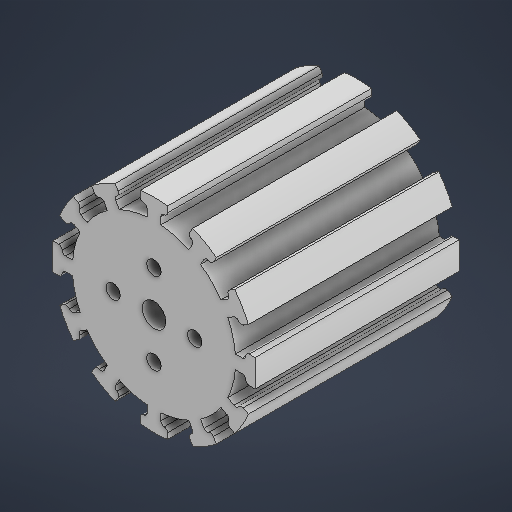
# Autodesk Inventor part: внутр сиськи
Saved by Autodesk Inventor 2025 (Build 290162000, 162)
## iProperties
Created: 2025-11-06
Part Number: внутр сиськи
Material: Типовые
Document SubType Name: Modeling
Designer: Phantom
Density: 1 g/cm^3
Appearance: По умолчанию
Author: Phantom
Autodesk Inventor part; units mm, degrees
ref_plane "YZ Plane" through (0, 0, 0) normal (1, 0, 0) x (0, 1, 0)
ref_plane "XZ Plane" through (0, 0, 0) normal (0, 1, 0) x (-1, 0, 0)
ref_plane "XY Plane" through (0, 0, 0) normal (0, 0, 1) x (1, 0, 0)
sketch "Эскиз1" plane through (0, 0, 0) normal (0, 0, 1) x (1, 0, 0)
  arc A0 (25.6449, 2.3551) -> (26.6449, 3.3551) centre (25.6449, 3.3551) ccw
  arc A1 (27.6449, 4.3551) -> (26.6449, 3.3551) centre (27.6449, 3.3551) ccw
  line L0 (27.6449, 4.3551) -> (29.3771, 4.3551)
  arc A2 (29.3771, -3.6449) -> (29.3771, 4.3551) centre (-0.3551, 0.3551) ccw
  line L1 (29.3771, -3.6449) -> (27.6449, -3.6449)
  arc A3 (26.6449, -2.6449) -> (27.6449, -3.6449) centre (27.6449, -2.6449) ccw
  arc A4 (26.6449, -2.6449) -> (25.6449, -1.6449) centre (25.6449, -2.6449) ccw
  line L2 (25.6449, -1.6449) -> (23.5615, -1.6449)
  arc A5 (21.3572, -9.8711) -> (23.5615, -1.6449) centre (-0.3551, 0.3551) ccw
  line L3 (21.3572, -9.8711) -> (23.1616, -10.9129)
  arc A6 (23.1616, -10.9129) -> (24.5276, -10.5469) centre (23.6616, -10.0469) ccw
  arc A7 (25.8936, -10.1808) -> (24.5276, -10.5469) centre (25.3936, -11.0469) ccw
  line L4 (25.8936, -10.1808) -> (27.3937, -11.0469)
  arc A8 (23.3937, -17.9751) -> (27.3937, -11.0469) centre (-0.3551, 0.3551) ccw
  line L5 (23.3937, -17.9751) -> (21.8936, -17.109)
  arc A9 (21.5276, -15.743) -> (21.8936, -17.109) centre (22.3936, -16.243) ccw
  arc A10 (21.5276, -15.743) -> (21.1616, -14.377) centre (20.6616, -15.243) ccw
  line L6 (21.1616, -14.377) -> (19.3572, -13.3352)
  arc A11 (13.3352, -19.3572) -> (19.3572, -13.3352) centre (-0.3551, 0.3551) ccw
  line L7 (13.3352, -19.3572) -> (14.377, -21.1616)
  arc A12 (14.377, -21.1616) -> (15.743, -21.5276) centre (15.243, -20.6616) ccw
  arc A13 (17.109, -21.8936) -> (15.743, -21.5276) centre (16.243, -22.3936) ccw
  line L8 (17.109, -21.8936) -> (17.9751, -23.3937)
  arc A14 (11.0469, -27.3937) -> (17.9751, -23.3937) centre (-0.3551, 0.3551) ccw
  line L9 (11.0469, -27.3937) -> (10.1808, -25.8936)
  arc A15 (10.5469, -24.5276) -> (10.1808, -25.8936) centre (11.0469, -25.3936) ccw
  arc A16 (10.5469, -24.5276) -> (10.9129, -23.1616) centre (10.0469, -23.6616) ccw
  line L10 (10.9129, -23.1616) -> (9.8711, -21.3572)
  arc A17 (1.6449, -23.5615) -> (9.8711, -21.3572) centre (-0.3551, 0.3551) ccw
  line L11 (1.6449, -23.5615) -> (1.6449, -25.6449)
  arc A18 (1.6449, -25.6449) -> (2.6449, -26.6449) centre (2.6449, -25.6449) ccw
  arc A19 (3.6449, -27.6449) -> (2.6449, -26.6449) centre (2.6449, -27.6449) ccw
  line L12 (3.6449, -27.6449) -> (3.6449, -29.3771)
  arc A20 (-4.3551, -29.3771) -> (3.6449, -29.3771) centre (-0.3551, 0.3551) ccw
  line L13 (-4.3551, -29.3771) -> (-4.3551, -27.6449)
  arc A21 (-3.3551, -26.6449) -> (-4.3551, -27.6449) centre (-3.3551, -27.6449) ccw
  arc A22 (-3.3551, -26.6449) -> (-2.3551, -25.6449) centre (-3.3551, -25.6449) ccw
  line L14 (-2.3551, -25.6449) -> (-2.3551, -23.5615)
  arc A23 (-10.5813, -21.3572) -> (-2.3551, -23.5615) centre (-0.3551, 0.3551) ccw
  line L15 (-10.5813, -21.3572) -> (-11.623, -23.1616)
  arc A24 (-11.623, -23.1616) -> (-11.257, -24.5276) centre (-10.757, -23.6616) ccw
  arc A25 (-10.891, -25.8936) -> (-11.257, -24.5276) centre (-11.757, -25.3936) ccw
  line L16 (-10.891, -25.8936) -> (-11.757, -27.3937)
  arc A26 (-18.6852, -23.3937) -> (-11.757, -27.3937) centre (-0.3551, 0.3551) ccw
  line L17 (-18.6852, -23.3937) -> (-17.8192, -21.8936)
  arc A27 (-16.4531, -21.5276) -> (-17.8192, -21.8936) centre (-16.9531, -22.3936) ccw
  arc A28 (-16.4531, -21.5276) -> (-15.0871, -21.1616) centre (-15.9531, -20.6616) ccw
  line L18 (-15.0871, -21.1616) -> (-14.0454, -19.3572)
  arc A29 (-20.0674, -13.3352) -> (-14.0454, -19.3572) centre (-0.3551, 0.3551) ccw
  line L19 (-20.0674, -13.3352) -> (-21.8717, -14.377)
  arc A30 (-21.8717, -14.377) -> (-22.2378, -15.743) centre (-21.3717, -15.243) ccw
  arc A31 (-22.6038, -17.109) -> (-22.2378, -15.743) centre (-23.1038, -16.243) ccw
  line L20 (-22.6038, -17.109) -> (-24.1039, -17.9751)
  arc A32 (-28.1039, -11.0469) -> (-24.1039, -17.9751) centre (-0.3551, 0.3551) ccw
  line L21 (-28.1039, -11.0469) -> (-26.6038, -10.1808)
  arc A33 (-25.2378, -10.5469) -> (-26.6038, -10.1808) centre (-26.1038, -11.0469) ccw
  arc A34 (-25.2378, -10.5469) -> (-23.8717, -10.9129) centre (-24.3717, -10.0469) ccw
  line L22 (-23.8717, -10.9129) -> (-22.0674, -9.8711)
  arc A35 (-24.2716, -1.6449) -> (-22.0674, -9.8711) centre (-0.3551, 0.3551) ccw
  line L23 (-24.2716, -1.6449) -> (-26.3551, -1.6449)
  arc A36 (-26.3551, -1.6449) -> (-27.3551, -2.6449) centre (-26.3551, -2.6449) ccw
  arc A37 (-28.3551, -3.6449) -> (-27.3551, -2.6449) centre (-28.3551, -2.6449) ccw
  line L24 (-28.3551, -3.6449) -> (-30.0872, -3.6449)
  arc A38 (-30.0872, 4.3551) -> (-30.0872, -3.6449) centre (-0.3551, 0.3551) ccw
  line L25 (-30.0872, 4.3551) -> (-28.3551, 4.3551)
  arc A39 (-27.3551, 3.3551) -> (-28.3551, 4.3551) centre (-28.3551, 3.3551) ccw
  arc A40 (-27.3551, 3.3551) -> (-26.3551, 2.3551) centre (-26.3551, 3.3551) ccw
  line L26 (-26.3551, 2.3551) -> (-24.2716, 2.3551)
  arc A41 (-22.0674, 10.5813) -> (-24.2716, 2.3551) centre (-0.3551, 0.3551) ccw
  line L27 (-22.0674, 10.5813) -> (-23.8717, 11.623)
  arc A42 (-23.8717, 11.623) -> (-25.2378, 11.257) centre (-24.3717, 10.757) ccw
  arc A43 (-26.6038, 10.891) -> (-25.2378, 11.257) centre (-26.1038, 11.757) ccw
  line L28 (-26.6038, 10.891) -> (-28.1039, 11.757)
  arc A44 (-24.1039, 18.6852) -> (-28.1039, 11.757) centre (-0.3551, 0.3551) ccw
  line L29 (-24.1039, 18.6852) -> (-22.6038, 17.8192)
  arc A45 (-22.2378, 16.4531) -> (-22.6038, 17.8192) centre (-23.1038, 16.9531) ccw
  arc A46 (-22.2378, 16.4531) -> (-21.8717, 15.0871) centre (-21.3717, 15.9531) ccw
  line L30 (-21.8717, 15.0871) -> (-20.0674, 14.0454)
  arc A47 (-14.0454, 20.0674) -> (-20.0674, 14.0454) centre (-0.3551, 0.3551) ccw
  line L31 (-14.0454, 20.0674) -> (-15.0871, 21.8717)
  arc A48 (-15.0871, 21.8717) -> (-16.4531, 22.2378) centre (-15.9531, 21.3717) ccw
  arc A49 (-17.8192, 22.6038) -> (-16.4531, 22.2378) centre (-16.9531, 23.1038) ccw
  line L32 (-17.8192, 22.6038) -> (-18.6852, 24.1039)
  arc A50 (-11.757, 28.1039) -> (-18.6852, 24.1039) centre (-0.3551, 0.3551) ccw
  line L33 (-11.757, 28.1039) -> (-10.891, 26.6038)
  arc A51 (-11.257, 25.2378) -> (-10.891, 26.6038) centre (-11.757, 26.1038) ccw
  arc A52 (-11.257, 25.2378) -> (-11.623, 23.8717) centre (-10.757, 24.3717) ccw
  line L34 (-11.623, 23.8717) -> (-10.5813, 22.0674)
  arc A53 (-2.3551, 24.2716) -> (-10.5813, 22.0674) centre (-0.3551, 0.3551) ccw
  line L35 (-2.3551, 24.2716) -> (-2.3551, 26.3551)
  arc A54 (-2.3551, 26.3551) -> (-3.3551, 27.3551) centre (-3.3551, 26.3551) ccw
  arc A55 (-4.3551, 28.3551) -> (-3.3551, 27.3551) centre (-3.3551, 28.3551) ccw
  line L36 (-4.3551, 28.3551) -> (-4.3551, 30.0872)
  arc A56 (3.6449, 30.0872) -> (-4.3551, 30.0872) centre (-0.3551, 0.3551) ccw
  line L37 (3.6449, 30.0872) -> (3.6449, 28.3551)
  arc A57 (2.6449, 27.3551) -> (3.6449, 28.3551) centre (2.6449, 28.3551) ccw
  arc A58 (2.6449, 27.3551) -> (1.6449, 26.3551) centre (2.6449, 26.3551) ccw
  line L38 (1.6449, 26.3551) -> (1.6449, 24.2716)
  arc A59 (9.8711, 22.0674) -> (1.6449, 24.2716) centre (-0.3551, 0.3551) ccw
  line L39 (9.8711, 22.0674) -> (10.9129, 23.8717)
  arc A60 (10.9129, 23.8717) -> (10.5469, 25.2378) centre (10.0469, 24.3717) ccw
  arc A61 (10.1808, 26.6038) -> (10.5469, 25.2378) centre (11.0469, 26.1038) ccw
  line L40 (10.1808, 26.6038) -> (11.0469, 28.1039)
  arc A62 (17.9751, 24.1039) -> (11.0469, 28.1039) centre (-0.3551, 0.3551) ccw
  line L41 (17.9751, 24.1039) -> (17.109, 22.6038)
  arc A63 (15.743, 22.2378) -> (17.109, 22.6038) centre (16.243, 23.1038) ccw
  arc A64 (15.743, 22.2378) -> (14.377, 21.8717) centre (15.243, 21.3717) ccw
  line L42 (14.377, 21.8717) -> (13.3352, 20.0674)
  arc A65 (19.3572, 14.0454) -> (13.3352, 20.0674) centre (-0.3551, 0.3551) ccw
  line L43 (19.3572, 14.0454) -> (21.1616, 15.0871)
  arc A66 (21.1616, 15.0871) -> (21.5276, 16.4531) centre (20.6616, 15.9531) ccw
  arc A67 (21.8936, 17.8192) -> (21.5276, 16.4531) centre (22.3936, 16.9531) ccw
  line L44 (21.8936, 17.8192) -> (23.3937, 18.6852)
  arc A68 (27.3937, 11.757) -> (23.3937, 18.6852) centre (-0.3551, 0.3551) ccw
  line L45 (27.3937, 11.757) -> (25.8936, 10.891)
  arc A69 (24.5276, 11.257) -> (25.8936, 10.891) centre (25.3936, 11.757) ccw
  arc A70 (24.5276, 11.257) -> (23.1616, 11.623) centre (23.6616, 10.757) ccw
  line L46 (23.1616, 11.623) -> (21.3572, 10.5813)
  arc A71 (23.5615, 2.3551) -> (21.3572, 10.5813) centre (-0.3551, 0.3551) ccw
  line L47 (23.5615, 2.3551) -> (25.6449, 2.3551)
  circle A72 centre (-0.3551, 0.3551) radius 3.5
  circle A73 centre (-0.3551, 0.3551) radius 12
  circle A74 centre (-0.3551, 12.3551) radius 4.5
  circle A75 centre (-12.3551, 0.3551) radius 4.5
  circle A76 centre (-0.3551, -11.6449) radius 4.5
  circle A77 centre (11.6449, 0.3551) radius 4.5
  point P0 (0, 0)
  point P1 (-0.3619, 0.2649)
  point P2 (0, 0.7101)
  point P3 (-0.7101, 0.7101)
  point P4 (-0.7101, 0)
  dimension "d1" = 24
  dimension "d0" = 7
  dimension "d2" = 9
  dimension "d5" = 360
  constraints: 144 point on circle, 96 end point, 77 centre point, 2 coincident, 1 vertical alignment, 15 other
  measures "d0" diameter of A72
  measures "d2" diameter of A74
extrude "Выдавливание1" add sketch "Эскиз1" along normal blind 60 contours A0 A1 L0 A2 L1 A3 A4 L2 A5 L3 A6 A7 L4 A8 L5 A9 A10 L6 A11 L7 A12 A13 L8 A14 L9 A15 A16 L10 A17 L11 A18 A19 L12 A20 L13 A21 A22 L14 A23 L15 A24 A25 L16 A26 L17 A27 A28 L18 A29 L19 A30 A31 L20 A32 L21 A33 A34 L22 A35 L23 A36 A37 L24 A38 L25 A39 A40 L26 A41 L27 A42 A43 L28 A44 L29 A45 A46 L30 A47 L31 A48 A49 L32 A50 L33 A51 A52 L34 A53 L35 A54 A55 L36 A56 L37 A57 A58 L38 A59 L39 A60 A61 L40 A62 L41 A63 A64 L42 A65 L43 A66 A67 L44 A68 L45 A69 A70 L46 A71 L47 | A77 A73 A76 A75 A74
sketch "Эскиз2" plane through (0, 0, 60) normal (0, 0, 1) x (1, 0, 0)
  line L0 (-4.3551, -27.6449) -> (-4.3551, -29.3771) projected
  arc A0 (-4.3551, -29.3771) -> (3.6449, -29.3771) centre (-0.3551, 0.3551) ccw projected
  line L1 (3.6449, -29.3771) -> (3.6449, -27.6449) projected
  arc A1 (3.6449, -27.6449) -> (2.6449, -26.6449) centre (2.6449, -27.6449) ccw projected
  arc A2 (1.6449, -25.6449) -> (2.6449, -26.6449) centre (2.6449, -25.6449) ccw projected
  line L2 (1.6449, -25.6449) -> (1.6449, -23.5615) projected
  arc A3 (1.6449, -23.5615) -> (9.8711, -21.3572) centre (-0.3551, 0.3551) ccw projected
  line L3 (9.8711, -21.3572) -> (10.9129, -23.1616) projected
  arc A4 (10.5469, -24.5276) -> (10.9129, -23.1616) centre (10.0469, -23.6616) ccw projected
  arc A5 (10.5469, -24.5276) -> (10.1808, -25.8936) centre (11.0469, -25.3936) ccw projected
  line L4 (10.1808, -25.8936) -> (11.0469, -27.3937) projected
  arc A6 (11.0469, -27.3937) -> (17.9751, -23.3937) centre (-0.3551, 0.3551) ccw projected
  line L5 (17.9751, -23.3937) -> (17.109, -21.8936) projected
  arc A7 (17.109, -21.8936) -> (15.743, -21.5276) centre (16.243, -22.3936) ccw projected
  arc A8 (14.377, -21.1616) -> (15.743, -21.5276) centre (15.243, -20.6616) ccw projected
  line L6 (14.377, -21.1616) -> (13.3352, -19.3572) projected
  arc A9 (13.3352, -19.3572) -> (19.3572, -13.3352) centre (-0.3551, 0.3551) ccw projected
  line L7 (19.3572, -13.3352) -> (21.1616, -14.377) projected
  arc A10 (21.5276, -15.743) -> (21.1616, -14.377) centre (20.6616, -15.243) ccw projected
  arc A11 (21.5276, -15.743) -> (21.8936, -17.109) centre (22.3936, -16.243) ccw projected
  line L8 (21.8936, -17.109) -> (23.3937, -17.9751) projected
  arc A12 (23.3937, -17.9751) -> (27.3937, -11.0469) centre (-0.3551, 0.3551) ccw projected
  line L9 (27.3937, -11.0469) -> (25.8936, -10.1808) projected
  arc A13 (25.8936, -10.1808) -> (24.5276, -10.5469) centre (25.3936, -11.0469) ccw projected
  arc A14 (23.1616, -10.9129) -> (24.5276, -10.5469) centre (23.6616, -10.0469) ccw projected
  line L10 (23.1616, -10.9129) -> (21.3572, -9.8711) projected
  arc A15 (21.3572, -9.8711) -> (23.5615, -1.6449) centre (-0.3551, 0.3551) ccw projected
  line L11 (23.5615, -1.6449) -> (25.6449, -1.6449) projected
  arc A16 (26.6449, -2.6449) -> (25.6449, -1.6449) centre (25.6449, -2.6449) ccw projected
  arc A17 (26.6449, -2.6449) -> (27.6449, -3.6449) centre (27.6449, -2.6449) ccw projected
  line L12 (27.6449, -3.6449) -> (29.3771, -3.6449) projected
  arc A18 (29.3771, -3.6449) -> (29.3771, 4.3551) centre (-0.3551, 0.3551) ccw projected
  line L13 (29.3771, 4.3551) -> (27.6449, 4.3551) projected
  arc A19 (27.6449, 4.3551) -> (26.6449, 3.3551) centre (27.6449, 3.3551) ccw projected
  arc A20 (25.6449, 2.3551) -> (26.6449, 3.3551) centre (25.6449, 3.3551) ccw projected
  line L14 (25.6449, 2.3551) -> (23.5615, 2.3551) projected
  arc A21 (23.5615, 2.3551) -> (21.3572, 10.5813) centre (-0.3551, 0.3551) ccw projected
  line L15 (21.3572, 10.5813) -> (23.1616, 11.623) projected
  arc A22 (24.5276, 11.257) -> (23.1616, 11.623) centre (23.6616, 10.757) ccw projected
  arc A23 (24.5276, 11.257) -> (25.8936, 10.891) centre (25.3936, 11.757) ccw projected
  line L16 (25.8936, 10.891) -> (27.3937, 11.757) projected
  arc A24 (27.3937, 11.757) -> (23.3937, 18.6852) centre (-0.3551, 0.3551) ccw projected
  line L17 (23.3937, 18.6852) -> (21.8936, 17.8192) projected
  arc A25 (21.8936, 17.8192) -> (21.5276, 16.4531) centre (22.3936, 16.9531) ccw projected
  arc A26 (21.1616, 15.0871) -> (21.5276, 16.4531) centre (20.6616, 15.9531) ccw projected
  line L18 (21.1616, 15.0871) -> (19.3572, 14.0454) projected
  arc A27 (19.3572, 14.0454) -> (13.3352, 20.0674) centre (-0.3551, 0.3551) ccw projected
  line L19 (13.3352, 20.0674) -> (14.377, 21.8717) projected
  arc A28 (15.743, 22.2378) -> (14.377, 21.8717) centre (15.243, 21.3717) ccw projected
  arc A29 (15.743, 22.2378) -> (17.109, 22.6038) centre (16.243, 23.1038) ccw projected
  line L20 (17.109, 22.6038) -> (17.9751, 24.1039) projected
  arc A30 (17.9751, 24.1039) -> (11.0469, 28.1039) centre (-0.3551, 0.3551) ccw projected
  line L21 (11.0469, 28.1039) -> (10.1808, 26.6038) projected
  arc A31 (10.1808, 26.6038) -> (10.5469, 25.2378) centre (11.0469, 26.1038) ccw projected
  arc A32 (10.9129, 23.8717) -> (10.5469, 25.2378) centre (10.0469, 24.3717) ccw projected
  line L22 (10.9129, 23.8717) -> (9.8711, 22.0674) projected
  arc A33 (9.8711, 22.0674) -> (1.6449, 24.2716) centre (-0.3551, 0.3551) ccw projected
  line L23 (1.6449, 24.2716) -> (1.6449, 26.3551) projected
  arc A34 (2.6449, 27.3551) -> (1.6449, 26.3551) centre (2.6449, 26.3551) ccw projected
  arc A35 (2.6449, 27.3551) -> (3.6449, 28.3551) centre (2.6449, 28.3551) ccw projected
  line L24 (3.6449, 28.3551) -> (3.6449, 30.0872) projected
  arc A36 (3.6449, 30.0872) -> (-4.3551, 30.0872) centre (-0.3551, 0.3551) ccw projected
  line L25 (-4.3551, 30.0872) -> (-4.3551, 28.3551) projected
  arc A37 (-4.3551, 28.3551) -> (-3.3551, 27.3551) centre (-3.3551, 28.3551) ccw projected
  arc A38 (-2.3551, 26.3551) -> (-3.3551, 27.3551) centre (-3.3551, 26.3551) ccw projected
  line L26 (-2.3551, 26.3551) -> (-2.3551, 24.2716) projected
  arc A39 (-2.3551, 24.2716) -> (-10.5813, 22.0674) centre (-0.3551, 0.3551) ccw projected
  line L27 (-10.5813, 22.0674) -> (-11.623, 23.8717) projected
  arc A40 (-11.257, 25.2378) -> (-11.623, 23.8717) centre (-10.757, 24.3717) ccw projected
  arc A41 (-11.257, 25.2378) -> (-10.891, 26.6038) centre (-11.757, 26.1038) ccw projected
  line L28 (-10.891, 26.6038) -> (-11.757, 28.1039) projected
  arc A42 (-11.757, 28.1039) -> (-18.6852, 24.1039) centre (-0.3551, 0.3551) ccw projected
  line L29 (-18.6852, 24.1039) -> (-17.8192, 22.6038) projected
  arc A43 (-17.8192, 22.6038) -> (-16.4531, 22.2378) centre (-16.9531, 23.1038) ccw projected
  arc A44 (-15.0871, 21.8717) -> (-16.4531, 22.2378) centre (-15.9531, 21.3717) ccw projected
  line L30 (-15.0871, 21.8717) -> (-14.0454, 20.0674) projected
  arc A45 (-14.0454, 20.0674) -> (-20.0674, 14.0454) centre (-0.3551, 0.3551) ccw projected
  line L31 (-20.0674, 14.0454) -> (-21.8717, 15.0871) projected
  arc A46 (-22.2378, 16.4531) -> (-21.8717, 15.0871) centre (-21.3717, 15.9531) ccw projected
  arc A47 (-22.2378, 16.4531) -> (-22.6038, 17.8192) centre (-23.1038, 16.9531) ccw projected
  line L32 (-22.6038, 17.8192) -> (-24.1039, 18.6852) projected
  arc A48 (-24.1039, 18.6852) -> (-28.1039, 11.757) centre (-0.3551, 0.3551) ccw projected
  line L33 (-28.1039, 11.757) -> (-26.6038, 10.891) projected
  arc A49 (-26.6038, 10.891) -> (-25.2378, 11.257) centre (-26.1038, 11.757) ccw projected
  arc A50 (-23.8717, 11.623) -> (-25.2378, 11.257) centre (-24.3717, 10.757) ccw projected
  line L34 (-23.8717, 11.623) -> (-22.0674, 10.5813) projected
  arc A51 (-22.0674, 10.5813) -> (-24.2716, 2.3551) centre (-0.3551, 0.3551) ccw projected
  line L35 (-24.2716, 2.3551) -> (-26.3551, 2.3551) projected
  arc A52 (-27.3551, 3.3551) -> (-26.3551, 2.3551) centre (-26.3551, 3.3551) ccw projected
  arc A53 (-27.3551, 3.3551) -> (-28.3551, 4.3551) centre (-28.3551, 3.3551) ccw projected
  line L36 (-28.3551, 4.3551) -> (-30.0872, 4.3551) projected
  arc A54 (-30.0872, 4.3551) -> (-30.0872, -3.6449) centre (-0.3551, 0.3551) ccw projected
  line L37 (-30.0872, -3.6449) -> (-28.3551, -3.6449) projected
  arc A55 (-28.3551, -3.6449) -> (-27.3551, -2.6449) centre (-28.3551, -2.6449) ccw projected
  arc A56 (-26.3551, -1.6449) -> (-27.3551, -2.6449) centre (-26.3551, -2.6449) ccw projected
  line L38 (-26.3551, -1.6449) -> (-24.2716, -1.6449) projected
  arc A57 (-24.2716, -1.6449) -> (-22.0674, -9.8711) centre (-0.3551, 0.3551) ccw projected
  line L39 (-22.0674, -9.8711) -> (-23.8717, -10.9129) projected
  arc A58 (-25.2378, -10.5469) -> (-23.8717, -10.9129) centre (-24.3717, -10.0469) ccw projected
  arc A59 (-25.2378, -10.5469) -> (-26.6038, -10.1808) centre (-26.1038, -11.0469) ccw projected
  line L40 (-26.6038, -10.1808) -> (-28.1039, -11.0469) projected
  arc A60 (-28.1039, -11.0469) -> (-24.1039, -17.9751) centre (-0.3551, 0.3551) ccw projected
  line L41 (-24.1039, -17.9751) -> (-22.6038, -17.109) projected
  arc A61 (-22.6038, -17.109) -> (-22.2378, -15.743) centre (-23.1038, -16.243) ccw projected
  arc A62 (-21.8717, -14.377) -> (-22.2378, -15.743) centre (-21.3717, -15.243) ccw projected
  line L42 (-21.8717, -14.377) -> (-20.0674, -13.3352) projected
  arc A63 (-20.0674, -13.3352) -> (-14.0454, -19.3572) centre (-0.3551, 0.3551) ccw projected
  line L43 (-14.0454, -19.3572) -> (-15.0871, -21.1616) projected
  arc A64 (-16.4531, -21.5276) -> (-15.0871, -21.1616) centre (-15.9531, -20.6616) ccw projected
  arc A65 (-16.4531, -21.5276) -> (-17.8192, -21.8936) centre (-16.9531, -22.3936) ccw projected
  line L44 (-17.8192, -21.8936) -> (-18.6852, -23.3937) projected
  arc A66 (-18.6852, -23.3937) -> (-11.757, -27.3937) centre (-0.3551, 0.3551) ccw projected
  line L45 (-11.757, -27.3937) -> (-10.891, -25.8936) projected
  arc A67 (-10.891, -25.8936) -> (-11.257, -24.5276) centre (-11.757, -25.3936) ccw projected
  arc A68 (-11.623, -23.1616) -> (-11.257, -24.5276) centre (-10.757, -23.6616) ccw projected
  line L46 (-11.623, -23.1616) -> (-10.5813, -21.3572) projected
  arc A69 (-10.5813, -21.3572) -> (-2.3551, -23.5615) centre (-0.3551, 0.3551) ccw projected
  line L47 (-2.3551, -23.5615) -> (-2.3551, -25.6449) projected
  arc A70 (-3.3551, -26.6449) -> (-2.3551, -25.6449) centre (-3.3551, -25.6449) ccw projected
  arc A71 (-3.3551, -26.6449) -> (-4.3551, -27.6449) centre (-3.3551, -27.6449) ccw projected
  circle A72 centre (11.6449, 0.3551) radius 4.5 projected
  circle A73 centre (-0.3551, 12.3551) radius 4.5 projected
  circle A74 centre (-12.3551, 0.3551) radius 4.5 projected
  circle A75 centre (-0.3551, 0.3551) radius 3.5 projected
  circle A76 centre (-0.3551, -11.6449) radius 4.5 projected
  circle A77 centre (-12.3551, 0.3551) radius 2.1
  circle A78 centre (-0.3551, 12.3551) radius 2.1
  circle A79 centre (11.6449, 0.3551) radius 2.1
  circle A80 centre (-0.3551, -11.6449) radius 2.1
  point P0 (0, 0)
  dimension "d9" = 4.2
  dimension "d10" = 4.2
  dimension "d11" = 4.2
  dimension "d12" = 4.2
  constraints: 4 centre point, 4 coincident
  measures "d9" diameter of A77
  measures "d10" diameter of A78
  measures "d11" diameter of A79
  measures "d12" diameter of A80
extrude "Выдавливание2" add sketch "Эскиз2" against normal blind 18 contours A71 A70 L47 A69 L46 A68 A67 L45 A66 L44 A65 A64 L43 A63 L42 A62 A61 L41 A60 L40 A59 A58 L39 A57 L38 A56 A55 L37 A54 L36 A53 A52 L35 A51 L34 A50 A49 L33 A48 L32 A47 A46 L31 A45 L30 A44 A43 L29 A42 L28 A41 A40 L27 A39 L26 A38 A37 L25 A36 L24 A35 A34 L23 A33 L22 A32 A31 L21 A30 L20 A29 A28 L19 A27 L18 A26 A25 L17 A24 L16 A23 A22 L15 A21 L14 A20 A19 L13 A18 L12 A17 A16 L11 A15 L10 A14 A13 L9 A12 L8 A11 A10 L7 A9 L6 A8 A7 L5 A6 L4 A5 A4 L3 A3 L2 A2 A1 L1 A0 L0 | A72 | A73 | A74 | A76
